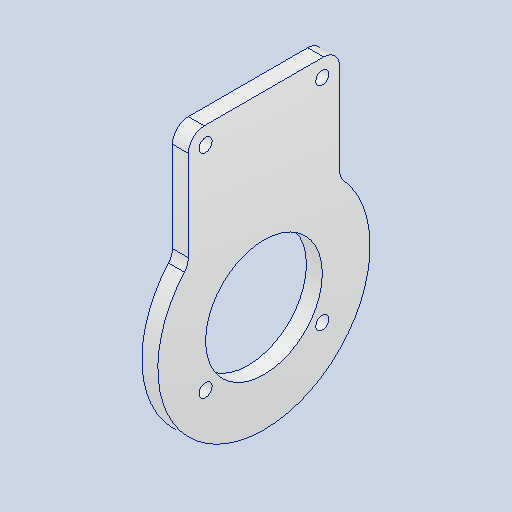
# Autodesk Inventor part: connectplate4
Saved by Autodesk Inventor 2024.3 (Build 283343010, 343A)
## iProperties
Created: 2025-06-29
Part Number: connectplate4
Material: アルミニウム 6061
Document SubType Name: Modeling
Designer: kshau
Density: 2.7 g/cm^3
Appearance: アルミニウム - フラット
Author: kshau
Autodesk Inventor part; units mm, degrees
ref_plane "YZ Plane" through (0, 0, 0) normal (1, 0, 0) x (0, 1, 0)
ref_plane "XZ Plane" through (0, 0, 0) normal (0, 1, 0) x (-1, 0, 0)
ref_plane "XY Plane" through (0, 0, 0) normal (0, 0, 1) x (1, 0, 0)
sketch "スケッチ1" plane through (0, 0, 0) normal (1, 0, 0) x (0, 1, 0)
  circle A0 centre (0, 0) radius 20
  line L0 (0, 0) -> (35.25, 0)
  line L1 (35.25, 0) -> (35.25, -14.25)
  line L2 (35.25, -14.25) -> (0, -14.25)
  line L3 (0, -14.25) -> (0, 0)
  line L4 (35.25, 0) -> (35.25, 14.25)
  line L5 (35.25, 14.25) -> (0, 14.25)
  point P0 (14.0334, 14.25)
  point P1 (14.0334, -14.25)
  dimension "d0" = 40
  dimension "d1" = 14.25
  dimension "d2" = 35.25
  constraints: 12 end point, 2 parallel, 2 symmetric about line, 1 centre point, 1 coincident, 1 horizontal, 1 perpendicular
  measures "d0" diameter of A0
  measures "d1" distance of L0.end L1.end
  measures "d2" distance of L1.end L2.end
extrude "押し出し1" add sketch "スケッチ1" along normal blind 3
sketch "スケッチ2" plane through (3, 0, 0) normal (1, 0, 0) x (0, 0, -1)
  line L0 (14.25, 35.25) -> (-14.25, 35.25) projected
  line L1 (-14.25, 35.25) -> (14.25, 35.25)
  line L2 (14.25, 35.25) -> (14.25, -11.25)
  line L3 (14.25, -11.25) -> (-14.25, -11.25)
  line L4 (-14.25, -11.25) -> (-14.25, 35.25)
  line L5 (-11, 32) -> (11, 32)
  line L6 (11, 32) -> (11, -8)
  line L7 (11, -8) -> (-11, -8)
  line L8 (-11, -8) -> (-11, 32)
  point P0 (0, 0)
  dimension "d5" = 46.5
  dimension "d6" = 3.25
  dimension "d7" = 3.25
  dimension "d8" = 3.25
  dimension "d9" = 3.25
  constraints: 16 end point, 4 coincident, 4 parallel, 2 horizontal, 2 perpendicular, 1 point on line
  measures "d5" distance of L1.end L2.end
  measures "d6" distance between parallel lines of L4 L8
  measures "d7" distance between parallel lines of L0 L5
  measures "d8" distance between parallel lines of L2 L6
  measures "d9" distance between parallel lines of L3 L7
hole "穴1" at (3, -8, 11) at (3, -8, -11) at (3, 32, -11) at (3, 32, 11) direction (-1, 0, 0) diameter 2.5 end through all
sketch "スケッチ3" plane through (0, 0, 0) normal (-1, 0, 0) x (0, 0, 1)
  circle A0 centre (0, 0) radius 11
  dimension "d17" = 22
  constraints: 1 centre point, 1 coincident
  measures "d17" diameter of A0
extrude "押し出し2" cut sketch "スケッチ3" against normal blind 3
fillet "フィレット1" radius 3 4 edges at (1.5, 35.25, 14.25) (1.5, 14.0334, 14.25) (1.5, 35.25, -14.25) (1.5, 14.0334, -14.25)
